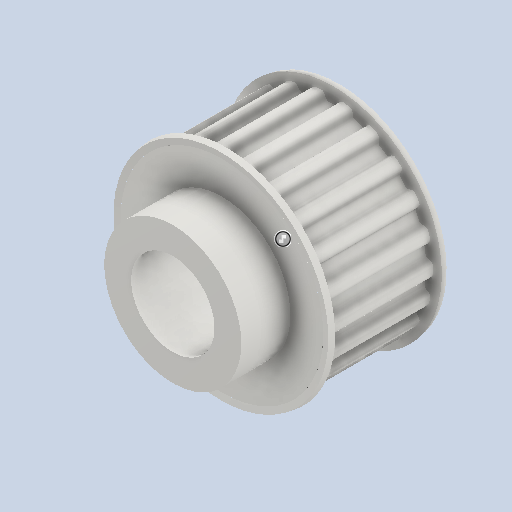
# Autodesk Inventor part: Synchroniczne koło pasowe2
Saved by Autodesk Inventor 2023 (Build 270158000, 158)
## iProperties
CustomPartVersion: 1
Created: 2023-04-25
Part Number: Synchroniczne koło pasowe2
Material: Steel
Document SubType Name: Modeling
Designer: krzys
Density: 7.85 g/cm^3
Appearance: Steel
Mass: 125.476 g
Surface Area: 65.0597 cm^2
Volume: 15.9843 cm^3
Author: krzys
Autodesk Inventor part; units mm, degrees
ref_plane "YZ Plane" through (0, 0, 0) normal (1, 0, 0) x (0, 1, 0)
ref_plane "XZ Plane" through (0, 0, 0) normal (0, 1, 0) x (-1, 0, 0)
ref_plane "XY Plane" through (0, 0, 0) normal (0, 0, 1) x (1, 0, 0)
sketch "Szkic koła pasowego" plane through (0, 0, 0) normal (0, 0, 1) x (1, 0, 0)
  circle A0 centre (0, 0) radius 17.507 construction
  circle A1 centre (0, 0) radius 17.007
  circle A2 centre (0, 0) radius 15.757
  line L0 (-1.4539, 16.9448) -> (-0.9, 15.757)
  line L1 (-0.9, 15.757) -> (0.9, 15.757)
  line L2 (0.9, 15.757) -> (1.4539, 16.9448)
  line L3 (0, 0) -> (0, 17.007) construction
  circle A3 centre (0, 0) radius 7
  circle A4 centre (0, 0) radius 11.5
  point P0 (0, 15.757)
  dimension "d0" = 35.0141
  dimension "d1" = 0.5
  dimension "d2" = 1.25
  dimension "d3" = 50
  dimension "d4" = 1.8
  dimension "d17" = 14
  dimension "d18" = 23
  constraints: 8 end point, 5 coincident, 4 centre point, 3 point on circle, 1 horizontal, 1 midpoint, 1 point on line, 1 vertical, 1 vertical alignment, 3 other
  measures "d0" diameter of A0
  measures "d1" radial gap between concentric circles of A0 A1
  measures "d3" angle of L2 L0
  measures "d4" distance of L0.end L1.end
  measures "d17" diameter of A3
  measures "d18" diameter of A4
extrude "Bryła podstawowa" add sketch "Szkic koła pasowego" along normal mid plane 17.5 contours A2 | A1 L0 L1 L2 | L2 L1 L0 A1 | A3 | A4
extrude "Ząb" cut sketch "Szkic koła pasowego" along normal through all both and the other way through all contours L2 L1 L0 A1 picked at (0, 16.5857)
fillet "Fillet" radius 0.4 2 edges at (0.9, 15.757, 0) (-0.9, 15.757, 0)
fillet "Fillet" radius 0.6 4 edges at (-1.4539, 16.9448, 4.375) (-1.4539, 16.9448, -4.375) (1.4539, 16.9448, 4.375) (1.4539, 16.9448, -4.375)
pattern_circular "Zęby" count 22 over 360 about axis through (0, 0, -10) along (0, 0, 1) of "Ząb", "Fillet"
pulley flange "Obrzeże lewe" diameter 34.0141 height 1.2 thickness 1 bend angle 10 centre (0, 0, -8.75) toward (0, 0, -1)
pulley flange "Obrzeże prawe" diameter 34.0141 height 1.2 thickness 1 bend angle 10 centre (0, 0, 8.75) toward (0, 0, 1)
extrude "Wyciągnięcie proste3" cut sketch "Szkic koła pasowego" along normal through all both and the other way through all contours A3
extrude "Wyciągnięcie proste4" add sketch "Szkic koła pasowego" along normal blind 18 contours A4
equation "\"d1\" = da_a"
equation "\"d2\" = da_hg"
equation "\"d3\" = 2 * da_fi"
equation "\"d4\" = da_bw"
equation "\"d5\" = da_bf"
equation "\"d7\" = da_bf"
equation "\"d9\" = da_rb"
equation "\"d10\" = da_rt"
equation "\"da_pb\" = 5"
equation "\"da_fi\" = 25deg"
equation "\"da_hg\" = 1.25"
equation "\"da_bw\" = 1.8"
equation "\"da_rb\" = 0.4"
equation "\"da_rt\" = 0.6"
equation "\"da_a\" = 0.5"
equation "\"da_bf\" = 17.5"
equation "\"da_wf\" = 1"
equation "\"da_hf\" = 1.2"
body "Solid1"
